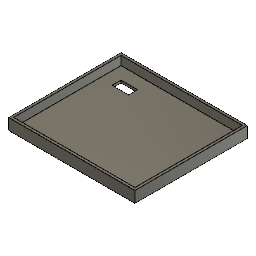
top v1 (Autodesk Fusion 360 design; units mm, degrees)
Autodesk Fusion 360 part; units mm, degrees
box "BoxPrimitive1" add length 89 width 100 height 2 placed x (0, 0, 1) y (1, 0, 0) z (0, 1, 0) at (0, 0, 0)
box "BoxPrimitive2" add length 89 width 2 height 7 placed x (0, 0, 1) y (1, 0, 0) z (0, 1, 0) at (0, 2, 0)
box "BoxPrimitive3" add length 89 width 2 height 7 placed x (0, 0, 1) y (1, 0, 0) z (0, 1, 0) at (98, 2, 0)
box "BoxPrimitive4" add length 2 width 96 height 7 placed x (0, 0, 1) y (1, 0, 0) z (0, 1, 0) at (2, 2, 0)
box "BoxPrimitive5" add length 2 width 96 height 7 placed x (0, 0, -1) y (-1, 0, 0) z (0, 1, 0) at (98, 2, 89)
box "BoxPrimitive6" cut length 7 width 13 height -2 placed x (0, 0, -1) y (-1, 0, 0) z (0, 1, 0) at (25, 2, 19)
